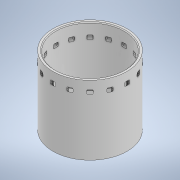
# Autodesk Inventor part: Box
Saved by Autodesk Inventor 2022.4 (Build 264492010, 492A)
## iProperties
Created: 2022-12-05
Part Number: Box
Material: Generic
Document SubType Name: Modeling
Designer: tmass
Density: 1 g/cm^3
Appearance: Default
Author: tmass
Autodesk Inventor part; units mm, degrees
ref_plane "XZ Plane" through (0, 0, 0) normal (0, 1, 0) x (-1, 0, 0)
ref_plane "XY Plane" through (0, 0, 0) normal (0, 0, 1) x (1, 0, 0)
sketch "Sketch1" plane through (0, 0, 0) normal (0, 1, 0) x (-1, 0, 0)
  circle A0 centre (0, 0) radius 42.025
  circle A1 centre (0, 0) radius 45.525
  dimension "d0" = 84.05
  dimension "d38" = 3.5
  constraints: 2 centre point, 2 coincident
  measures "d0" diameter of A0
  measures "d38" radial gap between concentric circles of A0 A1
extrude "Extrusion1" add sketch "Sketch1" along normal blind 85
sketch "Sketch2" plane through (0, 0, 0) normal (0, 0, 1) x (1, 0, 0)
  line L0 (45.525, 0) -> (45.525, 85) projected
  line L1 (42.025, 85) -> (42.025, 0) projected
  line L2 (45.525, 85) -> (-45.525, 85) projected
  line L3 (42.025, 71.5) -> (45.525, 75)
  line L4 (42.025, 66.5) -> (45.525, 70)
  line L5 (42.025, 71.5) -> (42.025, 66.5)
  line L6 (45.525, 70) -> (45.525, 75)
  line L7 (42.025, 71.5) -> (37.0637, 66.5387)
  line L8 (39.3318, 63.8068) -> (42.025, 66.5)
  line L9 (37.0637, 66.5387) -> (39.3318, 63.8068)
  point P0 (0, 0)
  point P1 (45.525, 70)
  dimension "d4" = 5
  dimension "d5" = 5
  dimension "d8" = 45
  dimension "d9" = 10
  constraints: 14 end point, 3 point on line, 2 parallel, 1 collinear
  measures "d4" distance of L4.start L3.start
  measures "d5" distance of L3.end L4.end
  measures "d8" angle of L1 L4
  measures "d9" distance of L3.end L0.end
extrude "Extrusion3" cut sketch "Sketch2" along normal mid plane 6 contours L4 L1 L3 L0 | L8 L9 L7 L1
fillet "Fillet1" radius 1 4 edges at (43.6719, 73.1469, 3) (43.6719, 73.1469, -3) (43.6719, 68.1469, 3) (43.6719, 68.1469, -3)
chamfer "Chamfer1" distance 1 angle 45 1 edges at (42.025, 85, 0)
pattern_circular "Circular Pattern2" count 16 over 360 about axis through (0, -10, 0) along (0, 1, 0) of "Fillet1", "Extrusion3"
ref_plane "Work Plane1" through (43, 0, 0) normal (1, 0, 0) x (0, 1, 0)
body "Solid1"
